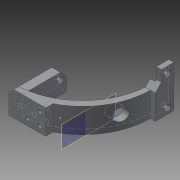
# Autodesk Inventor part: z-stepper support arm
Saved by Autodesk Inventor 2015 (Build 190159000, 159)
## iProperties
Created: 2019-01-12
Part Number: z-stepper support arm
Material: Generic
Document SubType Name: Modeling
Designer: Toby
Density: 1 g/cm^3
Appearance: Default
Author: Toby
Autodesk Inventor part; units mm, degrees
ref_plane "YZ Plane" through (0, 0, 0) normal (1, 0, 0) x (0, 1, 0)
ref_plane "XZ Plane" through (0, 0, 0) normal (0, 1, 0) x (-1, 0, 0)
ref_plane "XY Plane" through (0, 0, 0) normal (0, 0, 1) x (1, 0, 0)
sketch "Sketch1" plane through (0, 0, 0) normal (0, 0, 1) x (1, 0, 0)
  line L0 (-29.1667, 27.2576) -> (-22.1667, 27.2576)
  line L1 (-22.1667, 27.2576) -> (-22.1667, -12.7424)
  line L2 (-22.1667, -12.7424) -> (-29.1667, -12.7424)
  line L3 (-29.1667, -12.7424) -> (-29.1667, 27.2576)
  point P0 (0, 0)
  dimension "d0" = 7
  dimension "d1" = 40
  constraints: 8 end point, 2 parallel, 1 horizontal, 1 perpendicular
  measures "d0" distance of L0.start L0.end
  measures "d1" distance of L2.end L0.start
extrude "Extrusion1" add sketch "Sketch1" along normal blind 10
sketch "Sketch2" plane through (-22.1667, -12.7424, 0) normal (1, 0, 0) x (0, 0, -1)
  line L0 (-10, 0) -> (-10, 40) projected
  line L1 (0, 40) -> (-10, 40) projected
  point P0 (0, 12.7424)
  point P1 (-5, 35)
  dimension "d4" = 5
  dimension "d5" = 5
  measures "d4" distance from line of L0 point (-5, 35)
  measures "d5" distance from line of L1 point (-5, 35)
hole "Hole1" at (-22.1667, 22.2576, 5) direction (-1, 0, 0) diameter 3 depth 8 tip angle 118 countersink diameter 6 countersink angle 90
sketch "Sketch3" plane through (0, 0, 10) normal (0, 0, 1) x (1, 0, 0)
  line L0 (-29.1667, -12.7424) -> (30.8333, -12.7424)
  line L1 (30.8333, -12.7424) -> (30.8333, -8.7424)
  line L2 (30.8333, -8.7424) -> (-29.1667, -8.7424)
  line L3 (-29.1667, -8.7424) -> (-29.1667, -12.7424)
  line L4 (30.8333, -12.7424) -> (26.8333, -12.7424)
  line L5 (26.8333, -12.7424) -> (26.8333, 52.2576)
  line L6 (26.8333, 52.2576) -> (30.8333, 52.2576)
  line L7 (30.8333, 52.2576) -> (30.8333, -12.7424)
  point P0 (0, 0)
  dimension "d13" = 60
  dimension "d14" = 4
  dimension "d15" = 4
  dimension "d16" = 65
  constraints: 16 end point, 4 parallel, 2 horizontal, 2 perpendicular
  measures "d13" distance of L2.end L1.end
  measures "d14" distance of L1.end L0.end
  measures "d15" distance of L5.end L6.end
  measures "d16" distance of L4.end L5.end
extrude "Extrusion2" add sketch "Sketch3" against normal blind 10
sketch "Sketch4" plane through (30.8333, 52.2576, 10) normal (1, 0, 0) x (0, 0, -1)
  line L0 (16, -5) -> (-18, -5)
  line L1 (-18, -5) -> (-18, 5)
  line L2 (-18, 5) -> (16, 5)
  line L3 (16, 5) -> (16, -5)
  line L4 (0, 0) -> (10, 0) projected
  circle A0 centre (5, -30) radius 1.5 projected
  point P0 (10, -52.2576)
  dimension "d21" = 5
  dimension "d22" = 23
  dimension "d23" = 11
  dimension "d24" = 5
  constraints: 8 end point, 2 parallel, 1 coincident, 1 horizontal, 1 perpendicular
  measures "d21" distance between parallel lines of L2 L4
  measures "d22" distance from line of point (5, -30) L1
  measures "d23" distance from line of A0.centre L3
  measures "d24" distance between parallel lines of L4 L0
extrude "Extrusion3" add sketch "Sketch4" against normal blind 4 contours L0 L1 L2 L3
sketch "Sketch9" plane through (0, 0, 10) normal (0, 0, 1) x (1, 0, 0)
  line L0 (26.7106, 42.2576) -> (30.8333, 47.2576)
  line L1 (30.8333, 47.2576) -> (34.8333, 47.2576)
  line L2 (34.8333, 47.2576) -> (30.8333, 47.2576) projected
  line L3 (34.8333, 47.2576) -> (30.7106, 42.2576)
  line L4 (30.7106, 42.2576) -> (26.7106, 42.2576)
  point P0 (0, 0)
  constraints: 8 end point, 3 equal length
extrude "Extrusion8" add sketch "Sketch9" against normal blind 10
sketch "Sketch10" plane through (0, 0, 10) normal (0, 0, 1) x (1, 0, 0)
  line L0 (30.8333, 42.2576) -> (34.8333, 47.2576)
  line L1 (34.8333, 47.2576) -> (34.8333, 42.2576)
  line L2 (30.8333, 47.2576) -> (34.8333, 47.2576) projected
  line L3 (34.8333, 42.2576) -> (30.8333, 42.2576)
  point P0 (0, 0)
  constraints: 6 end point, 2 perpendicular
extrude "Extrusion9" cut sketch "Sketch10" against normal blind 10
sketch "Sketch12" plane through (0, 0, 0) normal (0, 0, -1) x (-1, 0, 0)
  point P0 (0, 0)
sketch "Sketch13" plane through (0, 0, 0) normal (0, 0, -1) x (-1, 0, 0)
  line L0 (29.1667, -12.7424) -> (-30.8333, -12.7424)
  line L1 (-30.8333, -12.7424) -> (-30.8333, -8.7424)
  line L2 (-30.8333, -8.7424) -> (29.1667, -8.7424)
  line L3 (29.1667, -8.7424) -> (29.1667, -12.7424)
  line L4 (-30.8333, 42.2576) -> (-26.8333, 42.2576)
  line L5 (-26.8333, 42.2576) -> (-26.8333, -12.7424)
  line L6 (-26.8333, -12.7424) -> (-30.8333, -12.7424)
  line L7 (-30.8333, -12.7424) -> (-30.8333, 42.2576)
  line L8 (-30.8333, 42.2576) -> (-34.8333, 47.2576)
  line L9 (-34.8333, 47.2576) -> (-30.8333, 42.2576) projected
  line L10 (-34.8333, 47.2576) -> (-30.8333, 47.2576)
  line L11 (-30.8333, 47.2576) -> (-26.8333, 42.2576)
  point P0 (0, 0)
  dimension "d53" = 60
  dimension "d54" = 4
  dimension "d55" = 4
  constraints: 22 end point, 6 equal length, 3 horizontal, 2 perpendicular, 1 point on line
  measures "d53" distance of L1.end L2.end
  measures "d54" distance of L0.end L1.end
  measures "d55" distance between parallel lines of L7 L5
extrude "Extrusion10" add sketch "Sketch13" along normal blind 6
sketch "Sketch14" plane through (0, 0, 10) normal (0, 0, 1) x (1, 0, 0)
  point P0 (0, 0)
sketch "Sketch15" plane through (0, 0, 10) normal (0, 0, 1) x (1, 0, 0)
  line L0 (-29.1667, -12.7424) -> (30.8333, -12.7424) projected
  line L1 (34.8333, 47.2576) -> (-22.1667, 47.2576)
  line L2 (-22.1667, 47.2576) -> (-22.1667, -12.7424)
  line L3 (-22.1667, -12.7424) -> (34.8333, -12.7424)
  line L4 (34.8333, -12.7424) -> (34.8333, 47.2576)
  line L5 (-22.1667, -8.7424) -> (-22.1667, 27.2576) projected
  point P0 (0, 0)
  constraints: 8 end point, 2 parallel, 1 collinear, 1 horizontal, 1 perpendicular, 1 point on line
extrude "Extrusion11" cut sketch "Sketch15" against normal blind 20
sketch "Sketch16" plane through (0, 0, -6) normal (0, 0, -1) x (-1, 0, 0)
  line L0 (29.1667, -12.7424) -> (-30.8333, -12.7424)
  line L1 (-30.8333, -12.7424) -> (-30.8333, -8.7424)
  line L2 (-30.8333, -8.7424) -> (29.1667, -8.7424)
  line L3 (29.1667, -8.7424) -> (29.1667, -12.7424)
  line L4 (-30.8333, 47.2576) -> (-26.8333, 47.2576)
  line L5 (-26.8333, 47.2576) -> (-26.8333, -12.7424)
  line L6 (-26.8333, -12.7424) -> (-30.8333, -12.7424)
  line L7 (-30.8333, -12.7424) -> (-30.8333, 47.2576)
  line L8 (-30.8333, 57.2576) -> (-30.8333, 47.2576) projected
  point P0 (0, 0)
  dimension "d60" = 4
  dimension "d61" = 4
  constraints: 16 end point, 4 parallel, 2 horizontal, 2 perpendicular, 1 collinear, 1 point on line
  measures "d60" distance of L5.end L6.end
  measures "d61" distance between parallel lines of L0 L2
extrude "Extrusion12" add sketch "Sketch16" against normal blind 20
sketch "Sketch17" plane through (0, 0, 0) normal (0, 0, -1) x (-1, 0, 0)
  line L0 (29.1667, 27.2576) -> (22.1667, 27.2576)
  line L1 (22.1667, 27.2576) -> (22.1667, -8.7424)
  line L2 (22.1667, -8.7424) -> (29.1667, -8.7424)
  line L3 (29.1667, -8.7424) -> (29.1667, 27.2576)
  point P0 (0, 0)
  constraints: 8 end point, 2 parallel, 1 horizontal, 1 perpendicular
extrude "Extrusion13" add sketch "Sketch17" along normal blind 6
sketch "Sketch18" plane through (30.8333, 47.2576, 28) normal (1, 0, 0) x (0, 0, -1)
  line L0 (0, 0) -> (0, 10) projected
  line L1 (34, 10) -> (34, -60) projected
  point P0 (28, -47.2576)
  point P1 (5, 5)
  point P2 (29, 5)
  dimension "d66" = 5
  dimension "d67" = 5
  measures "d66" distance from line of L0 point (5, 5)
  measures "d67" distance from line of L1 point (29, 5)
hole "Hole3" at (30.8333, 52.2576, 23) at (30.8333, 52.2576, -1) direction (-1, 0, 0) diameter 3 depth 8 tip angle 118 countersink diameter 6 countersink angle 90
fillet "Fillet4" radius 55 2 edges at (26.8333, -8.7424, 4) (30.8333, -12.7424, 4)
chamfer "Chamfer2" distance 4 angle 45 1 edges at (-29.1667, -10.7424, 14)
chamfer "Chamfer3" distance 5 angle 45 2 edges at (28.8333, 47.2576, 14) (-25.6667, 27.2576, 10)
sketch "Sketch19" plane through (30.8333, 47.2576, 28) normal (1, 0, 0) x (0, 0, -1)
  line L0 (0, 0) -> (34, 0)
  line L1 (34, 0) -> (34, 10)
  line L2 (34, 10) -> (0, 10)
  line L3 (0, 10) -> (0, 0)
  point P0 (28, -47.2576)
  constraints: 8 end point, 2 parallel, 1 horizontal, 1 perpendicular
extrude "Extrusion14" add sketch "Sketch19" along normal blind 4
sketch "Sketch20" plane through (30.8333, 42.2576, -6) normal (1, 0, 0) x (0, 0, -1)
  line L0 (-20, 0) -> (0, 0)
  line L1 (0, 0) -> (0, 5)
  line L2 (0, 5) -> (-20, 5)
  line L3 (-20, 5) -> (-20, 0)
  point P0 (-6, -42.2576)
  constraints: 8 end point, 2 parallel, 1 horizontal, 1 perpendicular
extrude "Extrusion15" add sketch "Sketch20" along normal blind 4
chamfer "Chamfer4" distance 5 angle 45 1 edges at (32.8333, 47.2576, 14)
sketch "Sketch21" plane through (26.8333, 47.2576, 28) normal (-1, 0, 0) x (0, 0, 1)
  line L0 (-34, -5) -> (-34, 10) projected
  line L1 (0, 10) -> (-34, 10)
  line L2 (-34, 10) -> (-34, 0)
  line L3 (-34, 0) -> (0, 0)
  line L4 (0, 0) -> (0, 10)
  line L5 (-9, 0) -> (0, 0) projected
  point P0 (-28, -47.2576)
  constraints: 8 end point, 2 parallel, 1 collinear, 1 horizontal, 1 perpendicular, 1 point on line
extrude "Extrusion16" cut sketch "Sketch21" against normal blind 4
chamfer "Chamfer5" distance 1 angle 45 1 edges at (26.8333, 47.2576, 6.5)
sketch "Sketch22" plane through (34.8333, 47.2576, 28) normal (1, 0, 0) x (0, 0, -1)
  line L0 (0, 10) -> (0, 0) projected
  line L1 (34, 10) -> (0, 10) projected
  line L2 (34, -5) -> (34, 10) projected
  point P0 (28, -47.2576)
  point P1 (5, 5)
  point P2 (29, 5)
  dimension "d94" = 5
  dimension "d95" = 5
  dimension "d96" = 5
  dimension "d97" = 5
  measures "d94" distance from line of L0 point (5, 5)
  measures "d95" distance from line of L1 point (5, 5)
  measures "d96" distance from line of L2 point (29, 5)
  measures "d97" distance from line of L1 point (29, 5)
hole "Hole4" at (34.8333, 52.2576, 23) at (34.8333, 52.2576, -1) direction (-1, 0, 0) diameter 3 depth 8 tip angle 118 countersink diameter 6 countersink angle 90
sketch "Sketch23" plane through (30.8333, 47.2576, 19) normal (0, 1, 0) x (1, 0, 0)
  line L0 (0, 0) -> (-4, 0)
  line L1 (-4, 0) -> (-4, 25)
  line L2 (-4, 25) -> (0, 25)
  line L3 (0, 25) -> (0, 0)
  point P0 (-30.8333, 19)
  constraints: 8 end point, 2 parallel, 1 horizontal, 1 perpendicular
extrude "Extrusion17" cut sketch "Sketch23" against normal blind 1
sketch "Sketch24" plane through (0, 0, 10) normal (0, 0, 1) x (1, 0, 0)
  point P0 (0, 0)
ref_plane "Work Plane1" through (15.8333, -12.7424, -6) normal (-1, 0, 0) x (0, 0, 1)
sketch "Sketch25" plane through (15.8333, -12.7424, -6) normal (-1, 0, 0) x (0, 0, 1)
  circle A0 centre (11, 35) radius 1.5 projected
  circle A1 centre (11, 35) radius 5
  point P0 (6, 12.7424)
  dimension "d108" = 10
  constraints: 2 coincident, 1 centre point
  measures "d108" diameter of A1
extrude "Extrusion18" cut sketch "Sketch25" against normal blind 50 contours A0 | A1
sketch "Sketch26" plane through (0, 0, 14) normal (0, 0, 1) x (1, 0, 0)
  line L0 (-24.1667, -12.7424) -> (0.8333, -12.7424)
  line L1 (0.8333, -12.7424) -> (0.8333, -8.7424)
  line L2 (0.8333, -8.7424) -> (-24.1667, -8.7424)
  line L3 (-24.1667, -8.7424) -> (-24.1667, -12.7424)
  line L4 (0.8333, -8.7424) -> (-4.1667, -8.7424)
  line L5 (-4.1667, -8.7424) -> (-4.1667, -5.7424)
  line L6 (-4.1667, -5.7424) -> (0.8333, -5.7424)
  line L7 (0.8333, -5.7424) -> (0.8333, -8.7424)
  point P0 (0, 0)
  dimension "d111" = 25
  dimension "d112" = 4
  dimension "d113" = 5
  dimension "d114" = 3
  constraints: 16 end point, 4 parallel, 2 horizontal, 2 perpendicular
  measures "d111" distance of L2.end L1.end
  measures "d112" distance of L1.end L0.end
  measures "d113" distance of L5.end L6.end
  measures "d114" distance between parallel lines of L2 L6
extrude "Extrusion19" add sketch "Sketch26" against normal blind 20
sketch "Sketch27" plane through (-29.1667, -12.7424, -6) normal (0, -1, 0) x (1, 0, 0)
  line L0 (55.8544, 20) -> (4, 20) projected
  line L1 (30, 20) -> (30, 0) projected
  line L2 (30, 0) -> (0, 0) projected
  point P0 (29.1667, 6)
  point P1 (25, 15)
  point P2 (25, 5)
  point P3 (15, 5)
  dimension "d117" = 5
  dimension "d118" = 5
  dimension "d119" = 5
  dimension "d120" = 5
  dimension "d121" = 10
  measures "d117" distance from line of L0 point (25, 15)
  measures "d118" distance from line of L1 point (25, 15)
  measures "d119" distance from line of L1 point (25, 5)
  measures "d120" distance from line of L2 point (25, 5)
  measures "d121" distance of point (25, 5) point (15, 5)
hole "Hole5" at (-4.1667, -12.7424, 9) at (-4.1667, -12.7424, -1) at (-14.1667, -12.7424, -1) direction (0, 1, 0) diameter 3 depth 6 tip angle 118
sketch "Sketch28" plane through (-29.1667, -12.7424, -6) normal (0, -1, 0) x (1, 0, 0)
  line L0 (8.7267, 12.1008) -> (6.2978, 10.7688)
  line L1 (6.2978, 10.7688) -> (8.7267, 9.2201)
  line L2 (8.7267, 9.2201) -> (8.7267, 12.1008)
  point P0 (29.1667, 6)
  constraints: 6 end point, 1 vertical
extrude "Extrusion20" cut sketch "Sketch28" against normal blind 1
body "Solid1"
